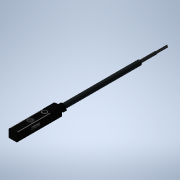
# Autodesk Inventor part: 8082090 SDBT-MSX-1L-NU-E-2.5-N-LE---(part)
Saved by Autodesk Inventor 2021 (Build 250183000, 183)
## iProperties
Created: 2025-06-16
Part Number: 8082090 SDBT-MSX-1L-NU-E-2.5-N-LE---(part)
Material: Generic
Catalog Web Link: www.cadenas.de
Description: SDBT-MSX_Schalter-Schalter
Vendor: FESTO
Document SubType Name: Modeling
Designer: psAdmin
Manufacturer: FESTO
Mass: 1.06499 g
Surface Area: 12.9885 cm^2
Volume: 1.06499 cm^3
Density: 1 g/cm^3
Appearance: PSOLRGB-175-175-175
Category: PARTsolutions
Company: FESTO
Title: 8082090 SDBT-MSX-1L-NU-E-2.5-N-LE---(part)
Author: Cadenas PARTsolutions
Comments: Schalter
PSOL_IDENT_0: {$CADENAS_DATA/23d-libs/festo/parts/s/sdbt/parts/sdbt_msx_schalter.prj},262 {VTYP=3D},{NB=8082090 SD
PSOL_IDENT_1: BT-MSX-1L-NU-E-2.5-N-LE---(part)},{LINA=8082090 SDBT-MSX-1L-NU-E-2.5-N-LE---(part)},{NN=SDBT-MSX_Sch
PSOL_IDENT_2: alter},{DATE=05.02.2025 08:22:47},{GEOMDATE=04.02.2025 20:10:00},{VERSION=},{LINEID=10},{WBVAR=SSZ,B
PSOL_IDENT_3: SA,SAD,LEI,LL,LEIT,ELA},{WBNUMERIC=}  {NB=8082090 SDBT-MSX-1L-NU-E-2.5-N-LE---(part)},{LINA=8082090
PSOL_IDENT_4: SDBT-MSX-1L-NU-E-2.5-N-LE---(part)},{KT=DUMMY},{TNR=8082090},{TYP=SDBT},{SSZ=MSX},{BSA=1L},{SAD=NU},
PSOL_IDENT_5: {LEI=E},{LL=2.5},{LEIT=N},{ELA=LE}
NB: 8082090 SDBT-MSX-1L-NU-E-2.5-N-LE---(part)
NN: SDBT-MSX_Schalter
NT: Schalter
NBSYN: $TNR. $TYP.-$SSZ.-$BSA.-$SAD.-$LEI.-$LL.-$LEIT.-$ELA.---(part)
LINA: 8082090 SDBT-MSX-1L-NU-E-2.5-N-LE---(part)
CATALOG: Festo
TNR: 8082090
TYP: SDBT
SSZ: MSX
BSA: 1L
SAD: NU
LEI: E
LL: 2.5
LEIT: N
ELA: LE
SUPPLIER: FESTO
ARTICLENO: 8082090 SDBT-MSX-1L-NU-E-2.5-N-LE---(part)
BOMINFO: 8082090 SDBT-MSX-1L-NU-E-2.5-N-LE---(part)
CREATOR: CADENAS GmbH
Autodesk Inventor part; units mm, degrees
sketch "Sketch_2" plane through (0, 0, 0) normal (0, 0, 1) x (1, 0, 0)
  line L0 (-2.525, 4.6576) -> (-2.525, 0)
  line L1 (-2.525, 0) -> (2.525, 0)
  line L2 (2.525, 0) -> (2.525, 4.6576)
  arc A0 (2.525, 4.6576) -> (2.3152, 4.9437) centre (2.225, 4.6576) ccw
  arc A1 (2.3152, 4.9437) -> (-2.3152, 4.9437) centre (0, -2.4) ccw
  arc A2 (-2.3152, 4.9437) -> (-2.525, 4.6576) centre (-2.225, 4.6576) ccw
  constraints: 6 end point, 6 point on circle, 3 centre point
extrude "Extrusion1" add sketch "Sketch_2" along normal blind 27.7
sketch "Sketch_5" plane through (0, 0, 0) normal (1, 0, 0) x (0, 1, 0)
  line L0 (5.2, 8.3) -> (5.8, 8.3)
  arc A0 (5.4292, 7.5227) -> (5.8, 8.3) centre (4.8, 8.3) ccw
  arc A1 (5.4292, 7.5227) -> (5.0748, 6.9262) centre (6.0583, 6.7455) ccw
  arc A2 (5.0748, 6.9262) -> (5.2, 8.3) centre (-2.4, 8.3) ccw
  line L1 (5.2, 8.3) -> (5.8, 8.3)
  constraints: 6 point on circle, 4 end point, 3 centre point
revolve "Revolution1" add sketch "Sketch_5" angle 360 about axis through (0, 5.2, 8.3) along (0, -1, 0)
sketch "Sketch_9" plane through (0, 5.5, 0) normal (0, 1, 0) x (1, 0, 0)
  circle A0 centre (0, -8.3) radius 1.5
  circle A1 centre (0, -8.3) radius 1.2
  constraints: 2 centre point
extrude "Extrusion2" cut sketch "Sketch_9" against normal blind 1
sketch "Sketch_10" plane through (0, 0, 8.3) normal (0, 0, 1) x (1, 0, 0)
  line L0 (-2, 5.015) -> (-2, 3)
  line L1 (-2, 3) -> (2, 3)
  line L2 (2, 3) -> (2, 5.015)
  arc A0 (2, 5.015) -> (-2, 5.015) centre (0, -2.4) ccw
  constraints: 6 end point, 2 point on circle, 1 centre point
extrude "Extrusion3" add sketch "Sketch_10" along normal mid plane 4
sketch "Sketch_16" plane through (0, 2, 0) normal (0, 1, 0) x (1, 0, 0)
  line L0 (-2.525, -15.175) -> (-2.525, -20.45)
  line L1 (-2.525, -20.45) -> (0.9243, -20.45)
  arc A0 (0.9243, -20.45) -> (1.1165, -20.3051) centre (0.9243, -20.25) ccw
  line L2 (1.1165, -20.3051) -> (1.3189, -19.5994)
  arc A1 (2.2802, -18.875) -> (1.3189, -19.5994) centre (2.2802, -19.875) ccw
  line L3 (2.2802, -18.875) -> (2.525, -18.875)
  line L4 (2.525, -18.875) -> (2.525, -13.6)
  line L5 (2.525, -13.6) -> (-0.9743, -13.6)
  arc A2 (-0.9743, -13.6) -> (-1.1665, -13.7449) centre (-0.9743, -13.8) ccw
  line L6 (-1.1665, -13.7449) -> (-1.3689, -14.4506)
  arc A3 (-2.3302, -15.175) -> (-1.3689, -14.4506) centre (-2.3302, -14.175) ccw
  line L7 (-2.3302, -15.175) -> (-2.525, -15.175)
  constraints: 16 end point, 8 point on circle, 4 centre point
extrude "Extrusion4" cut sketch "Sketch_16" along normal blind 1.85
sketch "Sketch_3" plane through (0, 0, 0) normal (1, 0, 0) x (0, 1, 0)
  line L0 (3.3, 17) -> (5.3, 17)
  line L1 (5.3, 17) -> (5.3, 15.225)
  line L2 (5.3, 15.225) -> (3.3, 15.225)
  line L3 (3.3, 15.225) -> (3.3, 17)
  line L4 (3.3, 17) -> (5.3, 17)
  constraints: 10 end point
revolve "Revolution2" cut sketch "Sketch_3" angle 360 about axis through (0, 3.3, 17) along (0, -1, 0)
sketch "Sketch_18" plane through (0, 2, 0) normal (0, 1, 0) x (1, 0, 0)
  arc A0 (-1.4406, -14.8959) -> (-2.3367, -18.021) centre (0, -17) ccw
  arc A1 (-2.3142, -18.359) -> (-2.3367, -18.021) centre (-2.7949, -18.2212) ccw
  line L0 (-2.3142, -18.359) -> (-2.492, -18.9788)
  arc A2 (-2.492, -18.9788) -> (-2.4725, -19.0706) centre (-2.3958, -19.0064) ccw
  arc A3 (-2.4725, -19.0706) -> (0.9996, -20.0662) centre (0, -17) ccw
  arc A4 (0.9996, -20.0662) -> (1.0647, -19.9987) centre (0.9686, -19.9711) ccw
  line L1 (1.0647, -19.9987) -> (1.2424, -19.3788)
  arc A5 (1.4406, -19.1041) -> (1.2424, -19.3788) centre (1.7231, -19.5167) ccw
  arc A6 (1.4406, -19.1041) -> (2.3367, -15.979) centre (0, -17) ccw
  arc A7 (2.3142, -15.641) -> (2.3367, -15.979) centre (2.7949, -15.7788) ccw
  line L2 (2.3142, -15.641) -> (2.492, -15.0212)
  arc A8 (2.492, -15.0212) -> (2.4725, -14.9294) centre (2.3958, -14.9936) ccw
  arc A9 (2.4725, -14.9294) -> (-0.9996, -13.9338) centre (0, -17) ccw
  arc A10 (-0.9996, -13.9338) -> (-1.0647, -14.0013) centre (-0.9686, -14.0289) ccw
  line L3 (-1.0647, -14.0013) -> (-1.2424, -14.6212)
  arc A11 (-1.4406, -14.8959) -> (-1.2424, -14.6212) centre (-1.7231, -14.4833) ccw
  circle A12 centre (0, -17) radius 1.75
  constraints: 24 point on circle, 13 centre point, 8 end point
extrude "Extrusion5" add sketch "Sketch_18" along normal blind 1
sketch "Sketch_19" plane through (0, 0, 0) normal (1, 0, 0) x (0, 0, -1)
  line L0 (-17, 2) -> (-17, 2.6393)
  line L1 (-17, 2.6393) -> (-16.25, 2.95)
  line L2 (-16.25, 2.95) -> (-16.25, 5.1)
  line L3 (-16.25, 5.1) -> (-15.3207, 5.1)
  line L4 (-15.3207, 5.1) -> (-15.25, 5.0293)
  line L5 (-15.25, 5.0293) -> (-15.25, 4.5207)
  line L6 (-15.25, 4.5207) -> (-15.3207, 4.45)
  line L7 (-15.3207, 4.45) -> (-15.55, 4.45)
  arc A0 (-15.55, 4.45) -> (-15.65, 4.35) centre (-15.55, 4.35) ccw
  line L8 (-15.65, 4.35) -> (-15.65, 3.95)
  arc A1 (-15.65, 3.95) -> (-15.55, 3.85) centre (-15.55, 3.95) ccw
  line L9 (-15.55, 3.85) -> (-15.25, 3.85)
  line L10 (-15.25, 3.85) -> (-15.25, 2.2145)
  line L11 (-15.25, 2.2145) -> (-15.4645, 2)
  line L12 (-15.4645, 2) -> (-17, 2)
  line L13 (-17, 2) -> (-17, 2.6393)
  constraints: 28 end point, 4 point on circle, 2 centre point
revolve "Revolution3" add sketch "Sketch_19" angle 360 about axis through (0, 2, 17) along (0, -1, 0)
thread "Thread1" size "M3.5x0.35" class "6g" standard "ISO Metric profile" length 0.9207
sketch "Sketch_21" plane through (0, 5.1, 0) normal (0, 1, 0) x (1, 0, 0)
  line L0 (-0.75, -17.433) -> (0, -17.866)
  line L1 (0, -17.866) -> (0.75, -17.433)
  line L2 (0.75, -17.433) -> (0.75, -16.567)
  line L3 (0.75, -16.567) -> (0, -16.134)
  line L4 (0, -16.134) -> (-0.75, -16.567)
  line L5 (-0.75, -16.567) -> (-0.75, -17.433)
  constraints: 12 end point
extrude "Extrusion6" cut sketch "Sketch_21" against normal blind 1.4
sketch "Sketch_1" plane through (0, 0, 0) normal (1, 0, 0) x (0, 1, 0)
  line L0 (2.35, -50) -> (2.35, 0)
  line L1 (2.35, 0) -> (4.35, 0)
  line L2 (4.35, 0) -> (4.35, -3)
  line L3 (4.35, -3) -> (3.8, -3)
  line L4 (3.8, -3) -> (3.8, -50)
  line L5 (3.8, -50) -> (2.35, -50)
  line L6 (2.35, -50) -> (2.35, 0)
  constraints: 14 end point
revolve "Revolution4" add sketch "Sketch_1" angle 360 about axis through (0, 2.35, -50) along (0, 0, -1)
sketch "Sketch_4" plane through (0, 0, -1.5) normal (0, 0, 1) x (1, 0, 0)
  line L0 (-3.05, 2.3616) -> (-3.05, 2.2678)
  arc A0 (-3.05, 2.2678) -> (-2.8847, 2.0709) centre (-2.85, 2.2678) ccw
  line L1 (-2.8847, 2.0709) -> (0, 1.5622)
  line L2 (0, 1.5622) -> (2.8847, 2.0709)
  arc A1 (2.8847, 2.0709) -> (3.05, 2.2678) centre (2.85, 2.2678) ccw
  line L3 (3.05, 2.2678) -> (3.05, 2.3616)
  arc A2 (3.05, 2.3616) -> (2.8153, 2.5586) centre (2.85, 2.3616) ccw
  line L4 (2.8153, 2.5586) -> (0, 2.0622)
  line L5 (0, 2.0622) -> (-2.8153, 2.5586)
  arc A3 (-2.8153, 2.5586) -> (-3.05, 2.3616) centre (-2.85, 2.3616) ccw
  constraints: 12 end point, 8 point on circle, 4 centre point
extrude "Extrusion7" add sketch "Sketch_4" along normal mid plane 2
sketch "Sketch_27" plane through (0, 0, -50) normal (0, 0, 1) x (1, 0, 0)
  circle A0 centre (-0.1, 2.9) radius 0.5
  constraints: 1 centre point
extrude "Extrusion8" add sketch "Sketch_27" against normal blind 10
sketch "Sketch_30" plane through (0, 0, -50) normal (0, 0, 1) x (1, 0, 0)
  circle A0 centre (-0.1, 2.9) radius 0.3
  constraints: 1 centre point
extrude "Extrusion9" add sketch "Sketch_30" against normal blind 17
sketch "Sketch_28" plane through (0, 0, -50) normal (0, 0, 1) x (1, 0, 0)
  circle A0 centre (-0.4464, 2.3) radius 0.5
  constraints: 1 centre point
extrude "Extrusion10" add sketch "Sketch_28" against normal blind 10
sketch "Sketch_31" plane through (0, 0, -50) normal (0, 0, 1) x (1, 0, 0)
  circle A0 centre (-0.4464, 2.3) radius 0.3
  constraints: 1 centre point
extrude "Extrusion11" add sketch "Sketch_31" against normal blind 17
sketch "Sketch_29" plane through (0, 0, -50) normal (0, 0, 1) x (1, 0, 0)
  circle A0 centre (0.2464, 2.3) radius 0.5
  constraints: 1 centre point
extrude "Extrusion12" add sketch "Sketch_29" against normal blind 10
sketch "Sketch_32" plane through (0, 0, -50) normal (0, 0, 1) x (1, 0, 0)
  circle A0 centre (0.2464, 2.3) radius 0.3
  constraints: 1 centre point
extrude "Extrusion13" add sketch "Sketch_32" against normal blind 17
sketch "Sketch_7" plane through (0, 0, 27) normal (0, 0, 1) x (1, 0, 0)
  arc A0 (2.375, 4.9035) -> (1.975, 5.0217) centre (0, -2.4) ccw
  line L0 (2.375, 4.9035) -> (2.375, 5.5)
  line L1 (2.375, 5.5) -> (1.975, 5.5)
  line L2 (1.975, 5.5) -> (1.975, 5.0217)
  constraints: 6 end point, 2 point on circle, 1 centre point
extrude "Extrusion14" cut sketch "Sketch_7" against normal blind 20
sketch "Sketch_8" plane through (0, 0, 27) normal (0, 0, 1) x (1, 0, 0)
  arc A0 (-1.975, 5.0217) -> (-2.375, 4.9035) centre (0, -2.4) ccw
  line L0 (-1.975, 5.0217) -> (-1.975, 5.5)
  line L1 (-1.975, 5.5) -> (-2.375, 5.5)
  line L2 (-2.375, 5.5) -> (-2.375, 4.9035)
  constraints: 6 end point, 2 point on circle, 1 centre point
extrude "Extrusion15" cut sketch "Sketch_8" against normal blind 20
ref_plane "ANBAU_XY" through (0, 2.35, -50) normal (0, 0, 1) x (1, 0, 0)
ref_plane "ANBAU_YZ" through (0, 2.35, -50) normal (1, 0, 0) x (0, 1, 0)
ref_plane "ANBAU_ZX" through (0, 2.35, -50) normal (0, 1, 0) x (0, 0, 1)
ref_plane "FDT_NUT_XY" through (0, 0, 27.7) normal (0, -1, 0) x (1, 0, 0)
ref_plane "FDT_NUT_YZ" through (0, 0, 27.7) normal (1, 0, 0) x (0, 0, 1)
ref_plane "FDT_NUT_ZX" through (0, 0, 27.7) normal (0, 0, 1) x (0, -1, 0)
ref_plane "IP_XY" through (0, 2.35, -50) normal (0, 0, -1) x (1, 0, 0)
ref_plane "IP_YZ" through (0, 2.35, -50) normal (1, 0, 0) x (0, -1, 0)
ref_plane "IP_ZX" through (0, 2.35, -50) normal (0, -1, 0) x (0, 0, -1)
body "Solid1"
